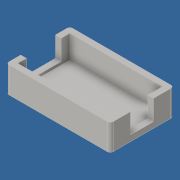
# Autodesk Inventor part: USB_case_A
Saved by Autodesk Inventor 2016 (Build 200138000, 138)
## iProperties
Created: 2017-06-14
Part Number: USB_case_A
Material: Generisch
Document SubType Name: Modeling
Designer: 4ndreas
Density: 1 g/cm^3
Appearance: Vorgabe
Author: 4ndreas
Autodesk Inventor part; units mm, degrees
ref_plane "YZ Plane" through (0, 0, 0) normal (1, 0, 0) x (0, 1, 0)
ref_plane "XZ Plane" through (0, 0, 0) normal (0, 1, 0) x (-1, 0, 0)
ref_plane "XY Plane" through (0, 0, 0) normal (0, 0, 1) x (1, 0, 0)
sketch "Skizze1" plane through (0, 0, 0) normal (0, 0, 1) x (1, 0, 0)
  line L0 (-16, -9) -> (16, -9)
  line L1 (16, -9) -> (16, 9)
  line L2 (16, 9) -> (-16, 9)
  line L3 (-16, 9) -> (-16, -9)
  line L4 (-16, -9) -> (16, 9) construction
  line L5 (16, -9) -> (-16, 9) construction
  line L6 (-18, 11) -> (18, 11)
  line L7 (18, 11) -> (18, -11)
  line L8 (18, -11) -> (-18, -11)
  line L9 (-18, -11) -> (-18, 11)
  point P0 (0, 0)
  dimension "d0" = 18
  dimension "d1" = 32
  dimension "d2" = 2
  constraints: 20 end point, 4 parallel, 2 midpoint, 2 perpendicular, 1 horizontal, 3 other
  measures "d0" distance between parallel lines of L0 L2
  measures "d1" distance between parallel lines of L3 L1
  measures "d2" distance between parallel lines of L2 L6
extrude "Extrusion1" add sketch "Skizze1" against normal blind 1 contours L3 L2 L1 L0 | L6 L7 L8 L9
extrude "Extrusion2" add sketch "Skizze1" along normal blind 6
sketch "Skizze2" plane through (0, 0, 6) normal (0, 0, 1) x (1, 0, 0)
  line L0 (-16, -9) -> (-16, 9) projected
  line L1 (-16, 9) -> (16, 9) projected
  line L2 (16, 9) -> (16, -9) projected
  line L3 (16, -9) -> (-16, -9) projected
  line L4 (18, 11) -> (-18, 11) projected
  line L5 (-18, 11) -> (-18, -11) projected
  line L6 (-18, -11) -> (18, -11) projected
  line L7 (18, -11) -> (18, 11) projected
  line L8 (-18, -6) -> (0, -6)
  line L9 (0, -6) -> (0, 6)
  line L10 (0, 6) -> (-18, 6)
  line L11 (-18, 6) -> (-18, -6)
  line L12 (-18, 11) -> (-18, -11) projected
  point P0 (0, 0)
  point P1 (0, 0)
  dimension "d7" = 12
  constraints: 8 end point, 2 parallel, 1 coincident, 1 collinear, 1 horizontal, 1 midpoint, 1 perpendicular
  measures "d7" distance between parallel lines of L8 L10
extrude "Extrusion3" cut sketch "Skizze2" against normal blind 5 contours L8 L5 L10 L0 | L0 L10 L9 L8
sketch "Skizze3" plane through (0, 0, 6) normal (0, 0, 1) x (1, 0, 0)
  line L0 (-18, 6) -> (-16, 6) projected
  line L1 (-16, 6) -> (-16, 9) projected
  line L2 (-16, 9) -> (16, 9) projected
  line L3 (16, 9) -> (16, -9) projected
  line L4 (16, -9) -> (-16, -9) projected
  line L5 (-16, -9) -> (-16, -6) projected
  line L6 (-16, -6) -> (-18, -6) projected
  line L7 (-18, -6) -> (-18, -11) projected
  line L8 (-18, -11) -> (18, -11) projected
  line L9 (18, -11) -> (18, 11) projected
  line L10 (18, 11) -> (-18, 11) projected
  line L11 (-18, 11) -> (-18, 6) projected
  line L12 (18, -4) -> (0, -4)
  line L13 (0, -4) -> (0, 4)
  line L14 (0, 4) -> (18, 4)
  line L15 (18, 4) -> (18, -4)
  point P0 (0, 0)
  point P1 (0, 0)
  point P2 (18, 0)
  dimension "d10" = 8
  constraints: 8 end point, 3 midpoint, 2 parallel, 1 coincident, 1 horizontal, 1 perpendicular
  measures "d10" distance between parallel lines of L14 L12
extrude "Extrusion4" cut sketch "Skizze3" against normal blind 5 contours L9 L12 L3 L14 | L3 L12 L13 L14
sketch "Skizze4" plane through (0, 0, 6) normal (0, 0, 1) x (1, 0, 0)
  line L0 (18, -4) -> (16, -4) projected
  line L1 (16, -4) -> (16, -9) projected
  line L2 (16, -9) -> (-16, -9) projected
  line L3 (-16, -9) -> (-16, -6) projected
  line L4 (-16, -6) -> (-18, -6) projected
  line L5 (-18, -6) -> (-18, -11) projected
  line L6 (-18, -11) -> (18, -11) projected
  line L7 (18, -11) -> (18, -4) projected
  line L8 (16, 4) -> (18, 4) projected
  line L9 (18, 4) -> (18, 11) projected
  line L10 (18, 11) -> (-18, 11) projected
  line L11 (-18, 11) -> (-18, 6) projected
  line L12 (-18, 6) -> (-16, 6) projected
  line L13 (-16, 6) -> (-16, 9) projected
  line L14 (-16, 9) -> (16, 9) projected
  line L15 (16, 9) -> (16, 4) projected
  point P0 (0, 0)
extrude "Extrusion5" add sketch "Skizze4" along normal blind 2
fillet "Rundung1" radius 1 4 edges at (18, 11, 3.5) (-18, 11, 3.5) (-18, -11, 3.5) (18, -11, 3.5)
